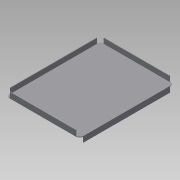
# Autodesk Inventor part: Cart_MID_SHELF
Saved by Autodesk Inventor 2015 (Build 190159000, 159)
## iProperties
Created: 2015-05-21
Part Number: Cart_MID_SHELF
Material: Generic
Document SubType Name: Modeling
Designer: Joe Sheldon
Density: 1 g/cm^3
Appearance: Default
Author: Joe Sheldon
Autodesk Inventor part; units mm, degrees
ref_plane "YZ Plane" through (0, 0, 0) normal (1, 0, 0) x (0, 1, 0)
ref_plane "XZ Plane" through (0, 0, 0) normal (0, 1, 0) x (-1, 0, 0)
ref_plane "XY Plane" through (0, 0, 0) normal (0, 0, 1) x (1, 0, 0)
sketch "Sketch1" plane through (0, 0, 0) normal (0, 1, 0) x (-1, 0, 0)
  line L0 (0, 0) -> (-361.95, 0)
  line L1 (-361.95, 0) -> (-361.95, -463.55)
  line L2 (-361.95, -463.55) -> (0, -463.55)
  line L3 (0, -463.55) -> (0, 0)
  dimension "d0" = 361.95
  dimension "d1" = 463.55
  constraints: 8 end point, 2 parallel, 1 horizontal, 1 perpendicular
  measures "d0" distance of L2.end L1.end
  measures "d1" distance of L1.end L0.end
extrude "Extrusion1" add sketch "Sketch1" along normal blind 2.794
fillet "Fillet1" radius 19.05 4 edges at (361.95, 1.397, 0) (361.95, 1.397, -463.55) (0, 1.397, -463.55) (0, 1.397, 0)
sketch "Sketch3" plane through (0, 0, 0) normal (0, -1, 0) x (1, 0, 0)
  line L0 (361.95, -19.05) -> (359.3341, -19.05)
  line L1 (359.3341, -19.05) -> (359.3341, -444.5)
  line L2 (359.3341, -444.5) -> (361.95, -444.5)
  line L3 (361.95, -444.5) -> (361.95, -19.05)
  point P0 (0, 0)
  constraints: 8 end point, 2 parallel, 1 horizontal, 1 perpendicular
extrude "Extrusion2" add sketch "Sketch3" along normal blind 25.4
sketch "Sketch4" plane through (0, 2.794, 0) normal (0, 1, 0) x (1, 0, 0)
  line L0 (19.05, 0) -> (342.8936, 0)
  line L1 (342.8936, 0) -> (342.8936, 2.7101)
  line L2 (342.8936, 2.7101) -> (19.05, 2.7101)
  line L3 (19.05, 2.7101) -> (19.05, 0)
  line L4 (0, 19.05) -> (2.9466, 19.05)
  line L5 (2.9466, 19.05) -> (2.9466, 444.7516)
  line L6 (2.9466, 444.7516) -> (0, 444.7516)
  line L7 (0, 444.7516) -> (0, 19.05)
  line L8 (342.9, 463.55) -> (19.05, 463.55)
  line L9 (19.05, 463.55) -> (19.05, 460.6098)
  line L10 (19.05, 460.6098) -> (342.9, 460.6098)
  line L11 (342.9, 460.6098) -> (342.9, 463.55)
  point P0 (0, 0)
  constraints: 24 end point, 6 parallel, 3 horizontal, 3 perpendicular
extrude "Extrusion3" add sketch "Sketch4" along normal blind 25.4
body "Solid1"
